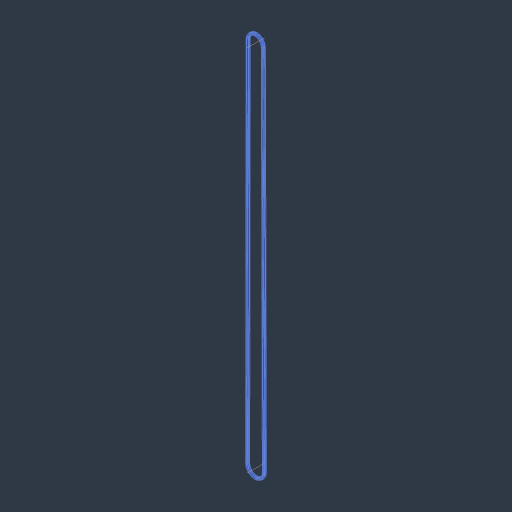
# Autodesk Inventor part: Roller Chain
Saved by Autodesk Inventor 2024.3 (Build 283343000, 343)
## iProperties
CustomPartVersion: 1
ILogicPurgeVersion: 0.0.0.0
OnSaveVersion: 3.4.3.0
OnSaveAssembly: COREAutomationManager
Created: 2025-01-30
Part Number: Roller Chain
Material: Generic
Document SubType Name: Modeling
Mfg Approved By: John.Thibert
Designer: John.Thibert
Density: 7.86109 g/cm^3
Appearance: Clear - Blue
Mass: 565.316 g
Surface Area: 726.344 cm^2
Volume: 71.9131 cm^3
ModelCat: Uncategorized
MaterialName: Generic
CN_MASS: 0.57
Author: John.Thibert
Autodesk Inventor part; units mm, degrees
ref_plane "Work Plane2" through (0, 0, 0) normal (-1, 0, 0) x (0, 0, 1)
ref_plane "Work Plane3" through (0.6898, -981.3217, 0) normal (0.1309701, 0.9913863, 0) x (0, 0, 1)
sketch "Path" plane through (0, 0, 0) normal (0, 0, 1) x (1, 0, 0)
  arc A0 (20.296, 0.0559) -> (-20.296, 0.0274) centre (0, 0) ccw
  arc A1 (-21.6198, -981.2916) -> (22.9994, -981.2603) centre (0.6898, -981.3217) ccw
  line L0 (-21.6198, -981.2916) -> (-20.296, 0.0274)
  line L1 (20.296, 0.0559) -> (22.9994, -981.2603)
  dimension "d31" = 5.9944
  constraints: 4 end point, 4 point on circle, 2 centre point
ref_plane "Section Plane" through (-20.296, 0.0274, 0) normal (-0.001349, -0.9999991, 0) x (0, 0, 1)
sketch "Section Sketch" plane through (-20.296, 0.0274, 0) normal (-0.001349, -0.9999991, 0) x (0, 0, 1)
  line L0 (-4.318, -1.1493) -> (4.318, -1.1493)
  line L1 (4.318, -1.1493) -> (4.318, 1.1493)
  line L2 (4.318, 1.1493) -> (-4.318, 1.1493)
  line L3 (-4.318, 1.1493) -> (-4.318, -1.1493)
  line L4 (-1.5875, -1.651) -> (1.5875, -1.651)
  line L5 (1.5875, -1.651) -> (1.5875, 1.651)
  line L6 (1.5875, 1.651) -> (-1.5875, 1.651)
  line L7 (-1.5875, 1.651) -> (-1.5875, -1.651)
  line L8 (-1.5875, 0) -> (1.5875, 0) construction
  line L9 (-3.1115, -2.9972) -> (-1.5875, -2.9972)
  line L10 (-1.5875, -2.9972) -> (-1.5875, 2.9972)
  line L11 (-1.5875, 2.9972) -> (-3.1115, 2.9972)
  line L12 (-3.1115, 2.9972) -> (-3.1115, -2.9972)
  line L13 (1.5875, -2.9972) -> (3.1115, -2.9972)
  line L14 (3.1115, -2.9972) -> (3.1115, 2.9972)
  line L15 (3.1115, 2.9972) -> (1.5875, 2.9972)
  line L16 (1.5875, 2.9972) -> (1.5875, -2.9972)
  line L17 (-4.318, 0) -> (4.318, 0) construction
  point P0 (0, 0)
  point P1 (0, 0)
  dimension "d21" = 2.2987
  dimension "d22" = 3.302
  dimension "d23" = 3.175
  dimension "d24" = 1.524
  dimension "d31" = 5.9944
  dimension "d32" = 8.636
  constraints: 36 end point, 8 midpoint, 8 parallel, 4 horizontal, 4 perpendicular, 3 collinear, 1 coincident, 1 other
  measures "d21" distance between parallel lines of L2 L0
  measures "d22" distance between parallel lines of L6 L4
  measures "d23" distance between parallel lines of L5 L7
  measures "d24" distance between parallel lines of L12 L10
  measures "d31" distance between parallel lines of L11 L9
  measures "d32" distance between parallel lines of L1 L3
sweep "Solid" add profiles "Section Sketch" path "Path"
pattern_of_one "Strand Pattern"
equation "\"d21\" = da_d2"
equation "\"d22\" = da_d1"
equation "\"d23\" = da_b1"
equation "\"d24\" = da_t1 + da_t2"
equation "\"d30\" = da_pt"
equation "\"da_p\" = 6.35"
equation "\"da_b1\" = 3.175"
equation "\"da_h2\" = 5.9944"
equation "\"da_h3\" = 5.207"
equation "\"da_d1\" = 3.302"
equation "\"da_d2\" = 2.2987"
equation "\"da_pt\" = 6.4008"
equation "\"da_b\" = 8.636"
equation "\"da_t1\" = 0.762"
equation "\"da_t2\" = 0.762"
body "Solid1"
